Autodesk Fusion 360 part; units mm, degrees
(part 4 of 5)
sketch "Sketch1" plane through (0, 0, 0) normal (0, 0, 1) x (1, 0, 0)
  line L0 (21.55, -50.4796) -> (21.55, -18.7607)
  line L1 (-21.55, -18.7607) -> (-21.55, -50.4796)
  circle A0 centre (15.25, -19.35) radius 2.95 construction
  circle A1 centre (-15.25, -19.35) radius 2.95 construction
  arc A2 (10.3384, 3) -> (6.0958, 1.2426) centre (10.3384, -3) ccw
  line L2 (-27.7114, -5.7461) -> (-23.2215, -12.9316)
  line L3 (29.5877, -66.4969) -> (23.2215, -56.3087)
  arc A3 (21.55, -50.4796) -> (23.2215, -56.3087) centre (32.55, -50.4796) ccw
  line L4 (4.8532, 0) -> (6.0958, 1.2426)
  circle A4 centre (15, -73.65) radius 2.95 construction
  arc A5 (4.5, -61) -> (8.3897, -57.7389) centre (6.3028, -59.2001) ccw
  line L5 (30.5, 15.05) -> (21.55, 15.05)
  arc A6 (8.0447, -57.2462) -> (6.6112, -56.5) centre (6.6112, -58.25) ccw
  line L6 (-4.5, -79.15) -> (4.5, -79.15) construction
  circle A7 centre (30.5, -79.95) radius 2 construction
  circle A8 centre (15.25, -49.85) radius 2.95 construction
  arc A9 (27.3521, -87.3046) -> (36.4601, -74.6136) centre (30.5, -79.95) ccw
  arc A10 (-8.3897, -57.7389) -> (-4.5, -61) centre (-6.3028, -59.2001) ccw
  arc A11 (-30.5, 15.05) -> (-33.9547, -0.1656) centre (-30.5, 7.05) ccw
  arc A12 (-6.0958, 1.2426) -> (-10.3384, 3) centre (-10.3384, -3) ccw
  line L7 (-27.3521, -87.3046) -> (-20.2, -84.2434)
  arc A13 (-31.6483, -69.2394) -> (-29.5877, -66.4969) centre (-46.5487, -55.8985) ccw
  line L8 (-13.5, 3) -> (-10.3384, 3)
  line L9 (-6.0958, 1.2426) -> (-4.8532, 0)
  line L10 (-31.6483, -69.2394) -> (-36.4601, -74.6136)
  arc A14 (15.1961, -0.0598) -> (13.5, 3) centre (13.5, 1) ccw
  arc A15 (19, 46.9161) -> (14.75, 54.55) centre (14.75, 49.55) ccw construction
  arc A16 (-36.4601, -74.6136) -> (-27.3521, -87.3046) centre (-30.5, -79.95) ccw
  circle A17 centre (-15.25, -49.85) radius 2.95 construction
  arc A18 (-6.6112, -56.5) -> (-8.0447, -57.2462) centre (-6.6112, -58.25) ccw
  line L11 (0.3197, 52.9873) -> (5.4482, 50.7517) construction
  arc A19 (2.7973, 58.6708) -> (-2.7973, 58.6708) centre (0, 52.254) ccw construction
  circle A20 centre (-15, -73.65) radius 2.95 construction
  line L12 (-23.2215, -56.3087) -> (-29.5877, -66.4969)
  arc A21 (18.55, 18.05) -> (21.55, 15.05) centre (21.55, 18.05) ccw construction
  arc A22 (-1.3481, 45.8161) -> (1.3481, 45.8161) centre (0, 47.9215) ccw construction
  arc A23 (33.9547, -0.1656) -> (30.5, 15.05) centre (30.5, 7.05) ccw
  line L13 (6.189, -12.7) -> (-6.189, -12.7) construction
  arc A24 (-13.5, 3) -> (-15.1961, -0.0598) centre (-13.5, 1) ccw
  circle A25 centre (15.25, -63.85) radius 1.5
  arc A26 (8.3, -79.15) -> (4.5, -79.15) centre (6.4, -82.51) ccw construction
  circle A27 centre (15.25, 8.95) radius 1.5
  circle A28 centre (-30.5, 7.05) radius 2 construction
  arc A29 (7.55, 40.0871) -> (5.7029, 41.0977) centre (6.35, 40.0871) ccw construction
  arc A30 (9.75, 29.95) -> (11.75, 29.95) centre (10.75, 29.95) ccw construction
  arc A31 (2.35, 33.9294) -> (3.3622, 32.0776) centre (4.55, 33.9294) ccw construction
  line L14 (10.9121, 55.1332) -> (2.7973, 58.6708) construction
  line L15 (-5.4482, 50.7517) -> (-0.3197, 52.9873) construction
  line L16 (9.75, 29.95) -> (9.75, 41.95) construction
  arc A32 (-13.7095, 54.55) -> (-10.9121, 55.1332) centre (-13.7095, 61.55) ccw construction
  line L17 (4.253, 25.5647) -> (8.8217, 22.262) construction
  line L18 (14.75, 54.55) -> (13.7095, 54.55) construction
  line L19 (6.43, 17.6256) -> (2.818, 20.406) construction
  line L20 (-2.7973, 58.6708) -> (-10.9121, 55.1332) construction
  circle A33 centre (-14.75, 49.55) radius 1.5 construction
  line L21 (9.65, 20.6411) -> (9.65, 19.2104) construction
  line L22 (2.35, 33.9294) -> (2.35, 37.7471) construction
  arc A34 (3.3637, 39.5999) -> (2.35, 37.7471) centre (4.55, 37.7471) ccw construction
  line L23 (-8.8217, 22.262) -> (-4.253, 25.5647) construction
  arc A35 (11.75, 41.95) -> (9.75, 41.95) centre (10.75, 41.95) ccw construction
  arc A36 (-13.55, 35.95) -> (-15.55, 35.95) centre (-14.55, 35.95) ccw construction
  line L24 (18.55, 18.05) -> (18.55, 45.3357) construction
  line L25 (-2.35, 24.5922) -> (-2.35, 21.3569) construction
  line L26 (13.55, 23.95) -> (13.55, 35.95) construction
  arc A37 (15.55, 35.95) -> (13.55, 35.95) centre (14.55, 35.95) ccw construction
  circle A38 centre (14.75, 49.55) radius 1.5 construction
  arc A39 (-2.818, 20.406) -> (-2.35, 21.3569) centre (-3.55, 21.3569) ccw construction
  line L27 (7.55, 40.0871) -> (7.55, 33.4162) construction
  arc A40 (5.6227, 48.5531) -> (5.4482, 50.7517) centre (4.9486, 49.6058) ccw construction
  arc A41 (-2.35, 37.7471) -> (-3.3637, 39.5999) centre (-4.55, 37.7471) ccw construction
  arc A42 (-3.3622, 32.0776) -> (-2.35, 33.9294) centre (-4.55, 33.9294) ccw construction
  arc A43 (4.1622, 31.5645) -> (7.55, 33.4162) centre (5.35, 33.4162) ccw construction
  line L28 (-11.75, 29.95) -> (-11.75, 41.95) construction
  line L29 (-2.818, 20.406) -> (-6.43, 17.6256) construction
  line L30 (-9.75, 41.95) -> (-9.75, 29.95) construction
  line L31 (4.1622, 31.5645) -> (3.3622, 32.0776) construction
  arc A44 (-14.75, 54.55) -> (-19, 46.9161) centre (-14.75, 49.55) ccw construction
  line L32 (11.75, 41.95) -> (11.75, 29.95) construction
  line L33 (-13.7095, 54.55) -> (-14.75, 54.55) construction
  line L34 (-15.55, 23.95) -> (-15.55, 35.95) construction
  arc A45 (-15.55, 23.95) -> (-13.55, 23.95) centre (-14.55, 23.95) ccw construction
  line L35 (5.6227, 48.5531) -> (1.3481, 45.8161) construction
  arc A46 (-7.55, 33.4162) -> (-4.1622, 31.5645) centre (-5.35, 33.4162) ccw construction
  line L36 (-9.65, 19.2104) -> (-9.65, 20.6411) construction
  arc A47 (-2.35, 24.5922) -> (-4.253, 25.5647) centre (-3.55, 24.5922) ccw construction
  line L37 (-1.3481, 45.8161) -> (-5.6227, 48.5531) construction
  arc A48 (-5.7029, 41.0977) -> (-7.55, 40.0871) centre (-6.35, 40.0871) ccw construction
  arc A49 (-18.55, 45.3357) -> (-19, 46.9161) centre (-21.55, 45.3357) ccw construction
  line L38 (-3.3622, 32.0776) -> (-4.1622, 31.5645) construction
  arc A50 (4.253, 25.5647) -> (2.35, 24.5922) centre (3.55, 24.5922) ccw construction
  arc A51 (0.3197, 52.9873) -> (-0.3197, 52.9873) centre (0, 52.254) ccw construction
  arc A52 (19, 46.9161) -> (18.55, 45.3357) centre (21.55, 45.3357) ccw construction
  line L39 (2.35, 21.3569) -> (2.35, 24.5922) construction
  arc A53 (10.9121, 55.1332) -> (13.7095, 54.55) centre (13.7095, 61.55) ccw construction
  line L40 (-13.55, 35.95) -> (-13.55, 23.95) construction
  arc A54 (13.55, 23.95) -> (15.55, 23.95) centre (14.55, 23.95) ccw construction
  line L41 (-2.35, 37.7471) -> (-2.35, 33.9294) construction
  line L42 (-7.55, 33.4162) -> (-7.55, 40.0871) construction
  arc A55 (9.65, 20.6411) -> (8.8217, 22.262) centre (7.65, 20.6411) ccw construction
  arc A56 (-5.4482, 50.7517) -> (-5.6227, 48.5531) centre (-4.9486, 49.6058) ccw construction
  arc A57 (2.35, 21.3569) -> (2.818, 20.406) centre (3.55, 21.3569) ccw construction
  arc A58 (-8.8217, 22.262) -> (-9.65, 20.6411) centre (-7.65, 20.6411) ccw construction
  line L43 (-5.7029, 41.0977) -> (-3.3637, 39.5999) construction
  line L44 (3.3637, 39.5999) -> (5.7029, 41.0977) construction
  line L45 (-18.55, 45.3357) -> (-18.55, 18.05) construction
  line L46 (15.55, 35.95) -> (15.55, 23.95) construction
  arc A59 (-9.75, 41.95) -> (-11.75, 41.95) centre (-10.75, 41.95) ccw construction
  arc A60 (-11.75, 29.95) -> (-9.75, 29.95) centre (-10.75, 29.95) ccw construction
  line L47 (4.5, -61) -> (-4.5, -61)
  arc A61 (6.43, 17.6256) -> (9.65, 19.2104) centre (7.65, 19.2104) ccw construction
  arc A62 (-9.65, 19.2104) -> (-6.43, 17.6256) centre (-7.65, 19.2104) ccw construction
  line L48 (36.4601, -74.6136) -> (31.6483, -69.2394)
  arc A63 (-21.55, 15.05) -> (-18.55, 18.05) centre (-21.55, 18.05) ccw construction
  line L49 (-6.6112, -56.5) -> (6.6112, -56.5)
  line L50 (-21.55, 15.05) -> (-30.5, 15.05)
  line L51 (8.0447, -57.2462) -> (8.3897, -57.7389)
  circle A64 centre (-15.25, 8.95) radius 1.5
  line L52 (8.3, -79.15) -> (27.3521, -87.3046) construction
  arc A65 (29.5877, -66.4969) -> (31.6483, -69.2394) centre (46.5487, -55.8985) ccw
  circle A66 centre (-30.5, -79.95) radius 2 construction
  line L53 (-8.3897, -57.7389) -> (-8.0447, -57.2462)
  arc A67 (-27.7114, -5.7461) -> (-33.9547, -0.1656) centre (-40.4322, -13.6949) ccw
  line L54 (10.3384, 3) -> (13.5, 3)
  arc A68 (23.2215, -12.9316) -> (21.55, -18.7607) centre (32.55, -18.7607) ccw
  arc A69 (-23.2215, -56.3087) -> (-21.55, -50.4796) centre (-32.55, -50.4796) ccw
  arc A70 (-4.5, -79.15) -> (-8.3, -79.15) centre (-6.4, -82.51) ccw construction
  arc A71 (33.9547, -0.1656) -> (27.7114, -5.7461) centre (40.4322, -13.6949) ccw
  arc A72 (-21.55, -18.7607) -> (-23.2215, -12.9316) centre (-32.55, -18.7607) ccw
  circle A73 centre (30.5, 7.05) radius 2 construction
  circle A74 centre (-15.25, -63.85) radius 1.5
  line L55 (-4.8532, 0) -> (4.8532, 0)
  line L56 (23.2215, -12.9316) -> (27.7114, -5.7461)
  line L57 (15.1961, -0.0598) -> (9.0119, -10.0491)
  circle A75 centre (-30.5, 7.05) radius 3.375
  circle A76 centre (30.5, 7.05) radius 3.375
  circle A77 centre (-30.5, -79.95) radius 3.375
  circle A78 centre (30.5, -79.95) radius 3.375
  circle A79 centre (-15.25, -19.35) radius 1.5
  circle A80 centre (15.25, -19.35) radius 1.5
  circle A81 centre (15.25, -49.85) radius 1.5
  circle A82 centre (-15.25, -49.85) radius 1.5
  line L58 (-15.25, -19.35) -> (15.25, -49.85) construction
  line L59 (-10, -24.6) -> (10, -24.6) construction
  line L60 (10, -24.6) -> (10, -44.6) construction
  line L61 (10, -44.6) -> (-10, -44.6) construction
  line L62 (-10, -44.6) -> (-10, -24.6) construction
  line L63 (-10, -24.6) -> (10, -44.6) construction
  line L64 (10, -24.6) -> (-10, -44.6) construction
  circle A83 centre (-10, -24.6) radius 1.5
  circle A84 centre (10, -24.6) radius 1.5
  circle A85 centre (10, -44.6) radius 1.5
  circle A86 centre (-10, -44.6) radius 1.5
  circle A87 centre (-15, -73.65) radius 1.5
  circle A88 centre (15, -73.65) radius 1.5
  line L65 (6.189, -11.4) -> (-6.189, -11.4)
  line L66 (0, 44.45) -> (0, -156.9165) construction
  spline S0 degree 5 poles (9.0119, -10.0491) (8.9382, -10.1683) (8.7794, -10.3902) (8.5077, -10.6735) (8.0875, -10.964) (7.4965, -11.2156) (6.9894, -11.3405) (6.5947, -11.3892) (6.3253, -11.4) (6.189, -11.4) knots 0 0 0 0 0 0 0.2 0.4 0.6 0.8 1 1 1 1 1 1
  line L67 (-15.1961, -0.0598) -> (-9.0119, -10.0491)
  spline S1 degree 5 poles (-9.0119, -10.0491) (-8.9382, -10.1683) (-8.7794, -10.3902) (-8.5077, -10.6735) (-8.0875, -10.964) (-7.4965, -11.2156) (-6.9894, -11.3405) (-6.5947, -11.3892) (-6.3253, -11.4) (-6.189, -11.4) knots 0 0 0 0 0 0 0.2 0.4 0.6 0.8 1 1 1 1 1 1
  line L68 (9.2055, -9.7365) -> (8.8184, -10.3617)
  line L69 (6.5567, -11.4) -> (5.8214, -11.4)
  line L70 (-9.2055, -9.7365) -> (-8.8184, -10.3617)
  line L71 (-6.5567, -11.4) -> (-5.8214, -11.4)
  line L72 (-5.45, -16.7) -> (5.45, -16.7)
  line L73 (5.45, -16.7) -> (5.45, -52.5)
  line L74 (5.45, -52.5) -> (-5.45, -52.5)
  line L75 (-5.45, -52.5) -> (-5.45, -16.7)
  line L76 (-5.45, -16.7) -> (5.45, -52.5) construction
  line L77 (5.45, -16.7) -> (-5.45, -52.5) construction
  line L78 (-5.45, -23.1541) -> (-4.312, -16.7)
  line L79 (-5.45, -23.1541) -> (0.7741, -23.1541) construction
  line L80 (-5.45, -46.0459) -> (-4.312, -52.5)
  line L81 (-5.45, -46.0459) -> (1.3736, -46.0459) construction
  line L82 (-4.312, -16.7) -> (-4.312, -52.5) construction
  line L83 (5.45, -46.0459) -> (4.312, -52.5)
  line L84 (5.45, -23.1541) -> (4.312, -16.7)
  line L85 (-20.2, -84.2434) -> (-20.2, -102.0248)
  line L86 (0, 18) -> (5, 18)
  line L87 (21.55, 15.05) -> (9.313, 15.05)
  arc A89 (5, 18) -> (9.313, 15.05) centre (9.313, 19.6778) ccw
  arc A90 (-9.313, 15.05) -> (-5, 18) centre (-9.313, 19.6778) ccw
  line L88 (-21.55, 15.05) -> (-9.313, 15.05)
  line L89 (0, 18) -> (-5, 18)
  line L90 (-15, -73.65) -> (-15, -103.65) construction
  circle A91 centre (-15, -103.65) radius 1.5
  circle A92 centre (-11.5, -118.65) radius 1.5
  circle A93 centre (-11.5, -118.65) radius 4.5
  line L91 (-15.7286, -120.1891) -> (-19.5733, -109.626)
  line L92 (-15.7286, -120.1891) -> (-5.1118, -120.1891) construction
  line L93 (-19.5733, -109.626) -> (-20.2, -102.0248)
  line L94 (0, -116) -> (-7.863, -116)
  line L95 (20.2, -84.2434) -> (20.2, -102.0248)
  circle A94 centre (15, -103.65) radius 1.5
  circle A95 centre (11.5, -118.65) radius 1.5
  line L96 (19.5733, -109.626) -> (20.2, -102.0248)
  line L97 (15.7286, -120.1891) -> (5.1118, -120.1891) construction
  line L98 (15.7286, -120.1891) -> (19.5733, -109.626)
  line L99 (0, -116) -> (7.863, -116)
  circle A96 centre (11.5, -118.65) radius 4.5
  line L100 (0, 44.45) -> (0, -156.9165) construction
  line L101 (27.3521, -87.3046) -> (20.2, -84.2434)
  point P0 (0, 44.45)
  point P1 (0, -34.6)
  point P2 (0, -34.6)
  point P3 (6.4, -82.51)
  point P4 (15, -103.65)
  dimension "d1" = 6.75
  dimension "d2" = 3
  dimension "d3" = 20
  dimension "d4" = 20
  dimension "d5" = 3
  dimension "d6" = 1.3
  dimension "d7" = 10.9
  dimension "d8" = 35.8
  dimension "d9" = 80
  dimension "d10" = 80
  dimension "d12" = 20.2
  dimension "d13" = 5
  dimension "d14" = 18
  dimension "d15" = 30
  dimension "d16" = 15
  dimension "d17" = 11.5
  dimension "d18" = 9
  dimension "d19" = 110
  dimension "d20" = 55
  constraint midpoint L55 origin
  constraint concentric A11 A75
  constraint concentric A23 A76
  constraint concentric A16 A77
  constraint concentric A7 A78
  constraint equal A77 A78
  constraint equal A76 A77
  constraint equal A75 A76
  constraint concentric A1 A79
  constraint concentric A0 A80
  constraint concentric A8 A81
  constraint concentric A17 A82
  constraint equal A81 A82
  constraint equal A80 A81
  constraint equal A79 A80
  constraint coincident A1.centre A79.centre
  constraint coincident A8.centre A81.centre
  constraint horizontal L59
  constraint perpendicular L59 L60
  constraint parallel L59 L61
  constraint parallel L60 L62
  constraint coincident L63 P2
  constraint coincident L64 P2
  constraint midpoint L58 P2
  constraint coincident L59.start L62.end
  constraint coincident L59.end L60.start
  constraint coincident L60.end L61.start
  constraint coincident L61.end L62.start
  constraint equal A85 A86
  constraint equal A84 A85
  constraint equal A83 A84
  constraint concentric A20 A87
  constraint concentric A4 A88
  constraint equal A87 A88
  constraint equal A81 A87
  constraint coincident P0 L66.start
  constraint perpendicular L59 L66
  constraint midpoint L57.end L68
  constraint midpoint L65.start L69
  constraint symmetric A14.start L66 A24.end
  constraint symmetric L57.end L66 L67.end
  constraint symmetric L65.start L66 L65.end
  constraint symmetric L66 L68.start L70.start
  constraint symmetric L66 L68.end L70.end
  constraint symmetric L66 L69.start L71.start
  constraint symmetric L66 L69.end L71.end
  constraint horizontal L72
  constraint perpendicular L72 L73
  constraint parallel L72 L74
  constraint parallel L73 L75
  constraint coincident L76 P2
  constraint coincident L77 P2
  constraint coincident P2 P1
  constraint horizontal L79
  constraint coincident L75 L78.start
  constraint horizontal L81
  constraint coincident L75 L80.start
  constraint coincident L74 L80.end
  constraint vertical L82
  constraint coincident L72 L78.end
  constraint symmetric L66 L78.start L84.start
  constraint symmetric L66 L78.end L84.end
  constraint symmetric L66 L80.start L83.start
  constraint symmetric L66 L80.end L83.end
  constraint parallel L66 L85
  constraint coincident L85 L7.end
  constraint coincident L66 L86.start
  constraint perpendicular L66 L86
  constraint tangent A21 L87
  constraint perpendicular L21 L87
  constraint horizontal L87
  constraint tangent L87 A89
  constraint symmetric L5.end L66 A63.start
  constraint symmetric L66 L86.start L89.start
  constraint symmetric L66 L86.end A90.end
  constraint symmetric L66 L87.end A90.start
  constraint symmetric L66 A89 A90
  constraint coincident A20.centre A87.centre
  constraint vertical L90
  constraint coincident L90.end A91.centre
  constraint equal A87 A91
  constraint equal A91 A92
  constraint concentric A92 A93
  constraint horizontal L92
  constraint coincident A93 L91.start
  constraint tangent A93 L91
  constraint coincident L66 L94.start
  constraint perpendicular L66 L94
  constraint coincident A93 L94.end
  constraint symmetric A70.centre L66 P3
  constraint symmetric P0 L66 L100.start
  constraint symmetric L100.end L66 L66.end
  constraint symmetric L66 L85.end L95.end
  constraint symmetric L66 L7.end L95.start
  constraint symmetric L66 L90.end P4
  constraint symmetric L66 A91 A94
  constraint symmetric L66 A92 A95
  constraint symmetric L66 A93 A96
  constraint symmetric L66 L91.start L97.start
  constraint symmetric L66 L91.end L96.start
  constraint symmetric L66 L92.end L97.end
  constraint symmetric L66 L94.start L99.start
  constraint symmetric L66 L94.end L99.end
  constraint symmetric L7.start L66 A9.start
  measures "d1" diameter of A75
  measures "d2" diameter of A79
  measures "d3" distance of L60.end L61.end
  measures "d4" distance of L59.end L60.end
  measures "d5" diameter of A83
  measures "d7" distance of L73.end L74.end
  measures "d8" distance of L72.end L73.end
  measures "d9" angle of L78 L79
  measures "d10" angle of L80 L81
  measures "d12" distance of L66 L85
  measures "d13" distance of L86.start L86.end
  measures "d14" distance of L55 L86
  measures "d15" distance of A20.centre L90.end
  measures "d16" vertical distance of L90.end A92.centre
  measures "d17" distance of L66 A92.centre
  measures "d18" diameter of A93
  measures "d19" angle of L91 L92
  measures "d20" distance of L47 L94
extrude "Extrude1" add sketch "Sketch1" along normal blind 2 contours L0 L1 L2 L3 A3 L5 A9 A11 L7 A13 L10 A16 L12 A23 L48 L50 A65 A67 A68 A69 A71 A72 L56 L85 L86 L87 A89 A90 L88 L89 A93 L91 L93 L94 L95 L96 L98 L99 A96 L101 | A96 | A93 | L72 L75 L78 | L72 L73 L84 | L74 L75 L80 | L73 L74 L83
fillet "Fillet1" radius 2 2 edges at (-20.2, -84.2434, 1) (20.2, -84.2434, 1)
fillet "Fillet2" radius 4 2 edges at (7.863, -116, 1) (-7.863, -116, 1)
fillet "Fillet3" radius 10 4 edges at (-19.5733, -109.626, 1) (-20.2, -102.0248, 1) (19.5733, -109.626, 1) (20.2, -102.0248, 1)
fillet "Fillet4" radius 1 4 edges at (-4.312, -16.7, 1) (4.312, -16.7, 1) (4.312, -52.5, 1) (-4.312, -52.5, 1)
fillet "Fillet5" radius 10 4 edges at (-5.45, -23.1541, 1) (5.45, -23.1541, 1) (5.45, -46.0459, 1) (-5.45, -46.0459, 1)
sketch "Sketch2" plane through (0, 0, 2) normal (0, 0, 1) x (1, 0, 0)
  arc A0 (20.1662, -102.4349) -> (20.2, -101.6132) centre (10.2, -101.6132) ccw
  line L0 (20.2, -101.6132) -> (20.2, -87.2749)
  arc A1 (22.987, -85.4363) -> (20.2, -87.2749) centre (22.2, -87.2749) ccw
  line L1 (22.987, -85.4363) -> (27.3521, -87.3046)
  arc A2 (27.3521, -87.3046) -> (36.4601, -74.6136) centre (30.5, -79.95) ccw
  line L2 (36.4601, -74.6136) -> (31.6483, -69.2394)
  arc A3 (29.5877, -66.4969) -> (31.6483, -69.2394) centre (46.5487, -55.8985) ccw
  line L3 (29.5877, -66.4969) -> (23.2215, -56.3087)
  arc A4 (21.55, -50.4796) -> (23.2215, -56.3087) centre (32.55, -50.4796) ccw
  line L4 (21.55, -50.4796) -> (21.55, -18.7607)
  arc A5 (23.2215, -12.9316) -> (21.55, -18.7607) centre (32.55, -18.7607) ccw
  line L5 (23.2215, -12.9316) -> (27.7114, -5.7461)
  arc A6 (33.9547, -0.1656) -> (27.7114, -5.7461) centre (40.4322, -13.6949) ccw
  arc A7 (33.9547, -0.1656) -> (30.5, 15.05) centre (30.5, 7.05) ccw
  line L6 (30.5, 15.05) -> (9.313, 15.05)
  arc A8 (5, 18) -> (9.313, 15.05) centre (9.313, 19.6778) ccw
  line L7 (5, 18) -> (-5, 18)
  arc A9 (-9.313, 15.05) -> (-5, 18) centre (-9.313, 19.6778) ccw
  line L8 (-9.313, 15.05) -> (-30.5, 15.05)
  arc A10 (-30.5, 15.05) -> (-33.9547, -0.1656) centre (-30.5, 7.05) ccw
  arc A11 (-27.7114, -5.7461) -> (-33.9547, -0.1656) centre (-40.4322, -13.6949) ccw
  line L9 (-27.7114, -5.7461) -> (-23.2215, -12.9316)
  arc A12 (-21.55, -18.7607) -> (-23.2215, -12.9316) centre (-32.55, -18.7607) ccw
  line L10 (-21.55, -18.7607) -> (-21.55, -50.4796)
  arc A13 (-23.2215, -56.3087) -> (-21.55, -50.4796) centre (-32.55, -50.4796) ccw
  line L11 (-23.2215, -56.3087) -> (-29.5877, -66.4969)
  arc A14 (-31.6483, -69.2394) -> (-29.5877, -66.4969) centre (-46.5487, -55.8985) ccw
  line L12 (-31.6483, -69.2394) -> (-36.4601, -74.6136)
  arc A15 (-36.4601, -74.6136) -> (-27.3521, -87.3046) centre (-30.5, -79.95) ccw
  line L13 (-27.3521, -87.3046) -> (-22.987, -85.4363)
  arc A16 (-20.2, -87.2749) -> (-22.987, -85.4363) centre (-22.2, -87.2749) ccw
  line L14 (-20.2, -87.2749) -> (-20.2, -101.6132)
  arc A17 (-20.2, -101.6132) -> (-20.1662, -102.4349) centre (-10.2, -101.6132) ccw
  line L15 (-20.1662, -102.4349) -> (-19.6835, -108.2886)
  arc A18 (-19.6835, -108.2886) -> (-19.1143, -110.8871) centre (-9.7173, -107.4669) ccw
  line L16 (-19.1143, -110.8871) -> (-15.7286, -120.1891)
  arc A19 (-15.7286, -120.1891) -> (-7.0571, -119.3647) centre (-11.5, -118.65) ccw
  arc A20 (-3.1079, -116) -> (-7.0571, -119.3647) centre (-3.1079, -120) ccw
  line L17 (-3.1079, -116) -> (3.1079, -116)
  arc A21 (7.0571, -119.3647) -> (3.1079, -116) centre (3.1079, -120) ccw
  arc A22 (7.0571, -119.3647) -> (15.7286, -120.1891) centre (11.5, -118.65) ccw
  line L18 (15.7286, -120.1891) -> (19.1143, -110.8871)
  arc A23 (19.1143, -110.8871) -> (19.6835, -108.2886) centre (9.7173, -107.4669) ccw
  line L19 (19.6835, -108.2886) -> (20.1662, -102.4349)
  circle A24 centre (-15.25, -49.85) radius 1.5
  arc A25 (-13.5, 3) -> (-15.1961, -0.0598) centre (-13.5, 1) ccw
  line L20 (-13.5, 3) -> (-10.3384, 3)
  arc A26 (-6.0958, 1.2426) -> (-10.3384, 3) centre (-10.3384, -3) ccw
  line L21 (-6.0958, 1.2426) -> (-4.8532, 0)
  line L22 (-4.8532, 0) -> (4.8532, 0)
  line L23 (4.8532, 0) -> (6.0958, 1.2426)
  arc A27 (10.3384, 3) -> (6.0958, 1.2426) centre (10.3384, -3) ccw
  line L24 (10.3384, 3) -> (13.5, 3)
  arc A28 (15.1961, -0.0598) -> (13.5, 3) centre (13.5, 1) ccw
  line L25 (15.1961, -0.0598) -> (9.0119, -10.0491)
  spline S0 degree 5 poles (9.0119, -10.0491) (8.9382, -10.1683) (8.7794, -10.3902) (8.5077, -10.6735) (8.0875, -10.964) (7.4965, -11.2156) (6.9894, -11.3405) (6.5947, -11.3892) (6.3253, -11.4) (6.189, -11.4) knots 0 0 0 0 0 0 0.2 0.4 0.6 0.8 1 1 1 1 1 1
  line L26 (6.189, -11.4) -> (-6.189, -11.4)
  spline S1 degree 5 poles (-6.189, -11.4) (-6.3253, -11.4) (-6.5947, -11.3892) (-6.9894, -11.3405) (-7.4965, -11.2156) (-8.0875, -10.964) (-8.5077, -10.6735) (-8.7794, -10.3902) (-8.9382, -10.1683) (-9.0119, -10.0491) knots -1 -1 -1 -1 -1 -1 -0.8 -0.6 -0.4 -0.2 0 0 0 0 0 0
  line L27 (-9.0119, -10.0491) -> (-15.1961, -0.0598)
  circle A29 centre (15.25, -49.85) radius 1.5
  circle A30 centre (15.25, -19.35) radius 1.5
  circle A31 centre (-15.25, -19.35) radius 1.5
  circle A32 centre (-15.25, -63.85) radius 1.5
  circle A33 centre (-30.5, 7.05) radius 3.375
  circle A34 centre (15, -73.65) radius 1.5
  circle A35 centre (-15, -73.65) radius 1.5
  circle A36 centre (-10, -44.6) radius 1.5
  circle A37 centre (10, -44.6) radius 1.5
  circle A38 centre (10, -24.6) radius 1.5
  circle A39 centre (-10, -24.6) radius 1.5
  line L28 (5.45, -24.029) -> (5.45, -45.171)
  arc A40 (5.2981, -46.9075) -> (5.45, -45.171) centre (-4.55, -45.171) ccw
  line L29 (5.2981, -46.9075) -> (4.4577, -51.6736)
  arc A41 (3.4729, -52.5) -> (4.4577, -51.6736) centre (3.4729, -51.5) ccw
  line L30 (3.4729, -52.5) -> (-3.4729, -52.5)
  arc A42 (-4.4577, -51.6736) -> (-3.4729, -52.5) centre (-3.4729, -51.5) ccw
  line L31 (-4.4577, -51.6736) -> (-5.2981, -46.9075)
  arc A43 (-5.45, -45.171) -> (-5.2981, -46.9075) centre (4.55, -45.171) ccw
  line L32 (-5.45, -45.171) -> (-5.45, -24.029)
  arc A44 (-5.2981, -22.2925) -> (-5.45, -24.029) centre (4.55, -24.029) ccw
  line L33 (-5.2981, -22.2925) -> (-4.4577, -17.5264)
  arc A45 (-3.4729, -16.7) -> (-4.4577, -17.5264) centre (-3.4729, -17.7) ccw
  line L34 (-3.4729, -16.7) -> (3.4729, -16.7)
  arc A46 (4.4577, -17.5264) -> (3.4729, -16.7) centre (3.4729, -17.7) ccw
  line L35 (4.4577, -17.5264) -> (5.2981, -22.2925)
  arc A47 (5.45, -24.029) -> (5.2981, -22.2925) centre (-4.55, -24.029) ccw
  circle A48 centre (30.5, 7.05) radius 3.375
  circle A49 centre (-30.5, -79.95) radius 3.375
  circle A50 centre (15.25, -63.85) radius 1.5
  circle A51 centre (15.25, 8.95) radius 1.5
  circle A52 centre (-15.25, 8.95) radius 1.5
  arc A53 (4.5, -61) -> (8.3897, -57.7389) centre (6.3028, -59.2001) ccw
  line L36 (4.5, -61) -> (-4.5, -61)
  arc A54 (-8.3897, -57.7389) -> (-4.5, -61) centre (-6.3028, -59.2001) ccw
  line L37 (-8.3897, -57.7389) -> (-8.0447, -57.2462)
  arc A55 (-6.6112, -56.5) -> (-8.0447, -57.2462) centre (-6.6112, -58.25) ccw
  line L38 (-6.6112, -56.5) -> (6.6112, -56.5)
  arc A56 (8.0447, -57.2462) -> (6.6112, -56.5) centre (6.6112, -58.25) ccw
  line L39 (8.0447, -57.2462) -> (8.3897, -57.7389)
  circle A57 centre (30.5, -79.95) radius 3.375
  circle A58 centre (11.5, -118.65) radius 1.5
  circle A59 centre (15, -103.65) radius 1.5
  circle A60 centre (-11.5, -118.65) radius 1.5
  circle A61 centre (-15, -103.65) radius 1.5
  line L40 (0, -116) -> (0, -61) construction
  line L41 (-15, -103.65) -> (-5.1101, -103.65) construction
  circle A62 centre (-10, -103.65) radius 1
  circle A63 centre (-10, -103.65) radius 3
  line L42 (-2.5, -103.3105) -> (-2.5, -113.346)
  line L43 (-2.5, -113.346) -> (-11.1856, -107.81)
  line L44 (-11.1856, -107.81) -> (-11.1856, -106.4058)
  line L45 (-2.5, -103.3105) -> (-4.5464, -101.7117)
  line L46 (-7, -103.65) -> (-7, -103.4617)
  line L47 (-5.25, -101.7117) -> (-4.5464, -101.7117)
  arc A64 (-5.25, -101.7117) -> (-7, -103.4617) centre (-5.25, -103.4617) ccw
  line L48 (-10, -103.65) -> (-10, -83.65) construction
  circle A65 centre (-10, -83.65) radius 1
  circle A66 centre (-10, -83.65) radius 3
  line L49 (-2.5, -84.401) -> (-2.5, -94.9628)
  line L50 (-2.5, -84.401) -> (-5.6804, -81.9162)
  line L51 (-2.5, -84.401) -> (1.142, -84.401) construction
  line L52 (-5.6804, -81.9162) -> (-7.3512, -85.0584)
  line L53 (-9.532, -86.6133) -> (-9.532, -90.422)
  line L54 (-9.532, -90.422) -> (-2.5, -94.9628)
  line L55 (10, -103.65) -> (10, -83.65) construction
  line L56 (2.5, -103.3105) -> (4.5464, -101.7117)
  line L57 (2.5, -103.3105) -> (2.5, -113.346)
  circle A67 centre (10, -103.65) radius 3
  line L58 (2.5, -113.346) -> (11.1856, -107.81)
  circle A68 centre (15, -103.65) radius 1.5
  line L59 (15, -103.65) -> (5.1101, -103.65) construction
  line L60 (11.1856, -107.81) -> (11.1856, -106.4058)
  line L61 (7, -103.65) -> (7, -103.4617)
  circle A69 centre (10, -103.65) radius 1
  line L62 (5.25, -101.7117) -> (4.5464, -101.7117)
  arc A70 (7, -103.4617) -> (5.25, -101.7117) centre (5.25, -103.4617) ccw
  line L63 (9.532, -90.422) -> (2.5, -94.9628)
  line L64 (2.5, -84.401) -> (2.5, -94.9628)
  line L65 (5.6804, -81.9162) -> (7.3512, -85.0584)
  line L66 (2.5, -84.401) -> (-1.142, -84.401) construction
  line L67 (2.5, -84.401) -> (5.6804, -81.9162)
  line L68 (9.532, -86.6133) -> (9.532, -90.422)
  circle A71 centre (10, -83.65) radius 3
  circle A72 centre (10, -83.65) radius 1
  point P0 (10.2, -101.6132)
  point P1 (9.7173, -107.4669)
  dimension "d33" = 2
  dimension "d34" = 5
  dimension "d35" = 6
  dimension "d36" = 2.5
  dimension "d37" = 1.75
  dimension "d38" = 20
  dimension "d39" = 2
  dimension "d40" = 6
  dimension "d41" = 2.5
  dimension "d42" = 128
  dimension "d43" = 142
  dimension "d44" = 80
  constraint midpoint L17 L40.start
  constraint midpoint L36 L40.end
  constraint coincident A61.centre L41.start
  constraint perpendicular L14 L41
  constraint coincident L41 A62.centre
  constraint concentric A62 A63
  constraint parallel L40 L42
  constraint coincident A63 L44.end
  constraint vertical L44
  constraint coincident L41 L46.start
  constraint coincident A63 L46.start
  constraint tangent A63 L46
  constraint perpendicular L46 L47
  constraint tangent L47 A64
  constraint tangent L46 A64
  constraint coincident A62.centre A63.centre
  constraint perpendicular L41 L48
  constraint coincident L48.end A65.centre
  constraint concentric A65 A66
  constraint vertical L49
  constraint horizontal L51
  constraint coincident A66 L52.end
  constraint tangent A66 L52
  constraint coincident A66 L53.start
  constraint parallel L48 L53
  constraint symmetric A17.centre L40 P0
  constraint symmetric A18.centre L40 P1
  constraint symmetric A61 L40 A68
  constraint symmetric L40 A61.centre A59.centre
  constraint symmetric L40 L41.end L59.end
  constraint symmetric L40 A62 A69
  constraint symmetric L40 A63 A67
  constraint symmetric L40 L42.start L56.start
  constraint symmetric L40 L42.end L57.end
  constraint symmetric L40 L43.end L58.end
  constraint symmetric L40 L44.end L60.end
  constraint symmetric L40 L45.end L56.end
  constraint symmetric L40 L46.start L61.start
  constraint symmetric L40 L47.start L62.start
  constraint symmetric L40 L46.end L61.end
  constraint symmetric L40 A64 A70
  constraint symmetric L40 A62.centre L55.start
  constraint symmetric L40 L48.end L55.end
  constraint symmetric L40 A65 A72
  constraint symmetric L40 A66 A71
  constraint symmetric L40 L49.start L64.start
  constraint symmetric L40 L49.end L63.end
  constraint symmetric L40 L50.end L65.start
  constraint symmetric L40 L51.end L66.end
  constraint symmetric L40 L52.end L65.end
  constraint symmetric L40 L53.start L68.start
  constraint symmetric L40 L53.end L63.start
  measures "d33" diameter of A62
  measures "d34" distance of A61.centre A62.centre
  measures "d35" diameter of A63
  measures "d36" distance of L40 L42
  measures "d37" radius of A64
  measures "d38" distance of A62.centre L48.end
  measures "d39" diameter of A65
  measures "d40" diameter of A66
  measures "d41" distance of L40 L49
  measures "d42" angle of L42 L45
  measures "d43" angle of L50 L51
  measures "d44" angle of L50 L52
extrude "Extrude2" cut sketch "Sketch2" against normal blind 2 contours A62 | A63 L42 L43 L44 L45 L46 L47 A64 | A65 | A66 L49 L50 L52 L53 L54 | L56 L57 A67 L58 L60 L61 L62 A70 | A69 | L63 L64 L65 L67 L68 A71 | A72
fillet "Fillet6" radius 2 4 edges at (-5.6804, -81.9162, 1) (-2.5, -84.401, 1) (2.5, -84.401, 1) (5.6804, -81.9162, 1)
fillet "Fillet7" radius 1 4 edges at (-2.5, -94.9628, 1) (2.5, -94.9628, 1) (2.5, -113.346, 1) (-2.5, -113.346, 1)
fillet "Fillet8" radius 1.5 4 edges at (-4.5464, -101.7117, 1) (-2.5, -103.3105, 1) (4.5464, -101.7117, 1) (2.5, -103.3105, 1)
fillet "Fillet9" radius 1.5 4 edges at (-9.532, -90.422, 1) (-9.532, -86.6133, 1) (9.532, -90.422, 1) (9.532, -86.6133, 1)
fillet "Fillet10" radius 1.5 4 edges at (11.1856, -107.81, 1) (11.1856, -106.4058, 1) (-11.1856, -107.81, 1) (-11.1856, -106.4058, 1)
sketch "Sketch3" plane through (0, 0, 2) normal (0, 0, 1) x (1, 0, 0)
  circle A0 centre (10, -103.65) radius 1
  circle A1 centre (-10, -83.65) radius 1
  line L0 (-5.25, -101.7117) -> (-5.0629, -101.7117)
  arc A2 (-4.1394, -102.0297) -> (-5.0629, -101.7117) centre (-5.0629, -103.2117) ccw
  line L1 (-4.1394, -102.0297) -> (-3.0765, -102.8601)
  arc A3 (-2.5, -104.0421) -> (-3.0765, -102.8601) centre (-4, -104.0421) ccw
  line L2 (-2.5, -104.0421) -> (-2.5, -111.5227)
  arc A4 (-4.0375, -112.366) -> (-2.5, -111.5227) centre (-3.5, -111.5227) ccw
  line L3 (-4.0375, -112.366) -> (-9.1581, -109.1022)
  arc A5 (-8.9013, -106.4416) -> (-9.1581, -109.1022) centre (-8.3519, -107.8373) ccw
  arc A6 (-8.9013, -106.4416) -> (-7, -103.65) centre (-10, -103.65) ccw
  line L4 (-7, -103.65) -> (-7, -103.4617)
  arc A7 (-5.25, -101.7117) -> (-7, -103.4617) centre (-5.25, -103.4617) ccw
  line L5 (8.8457, -90.8652) -> (4.0425, -93.9668)
  arc A8 (2.5, -93.1267) -> (4.0425, -93.9668) centre (3.5, -93.1267) ccw
  line L6 (2.5, -93.1267) -> (2.5, -85.3765)
  arc A9 (3.2687, -83.8004) -> (2.5, -85.3765) centre (4.5, -85.3765) ccw
  line L7 (3.2687, -83.8004) -> (3.8022, -83.3836)
  arc A10 (6.7994, -84.0207) -> (3.8022, -83.3836) centre (5.0335, -84.9596) ccw
  line L8 (6.7994, -84.0207) -> (7.3512, -85.0584)
  arc A11 (7.3512, -85.0584) -> (8.688, -86.3479) centre (10, -83.65) ccw
  arc A12 (9.532, -87.6968) -> (8.688, -86.3479) centre (8.032, -87.6968) ccw
  line L9 (9.532, -87.6968) -> (9.532, -89.6051)
  arc A13 (8.8457, -90.8652) -> (9.532, -89.6051) centre (8.032, -89.6051) ccw
  arc A14 (9.1581, -109.1022) -> (8.9013, -106.4416) centre (8.3519, -107.8373) ccw
  line L10 (9.1581, -109.1022) -> (4.0375, -112.366)
  arc A15 (2.5, -111.5227) -> (4.0375, -112.366) centre (3.5, -111.5227) ccw
  line L11 (2.5, -111.5227) -> (2.5, -104.0421)
  arc A16 (3.0765, -102.8601) -> (2.5, -104.0421) centre (4, -104.0421) ccw
  line L12 (3.0765, -102.8601) -> (4.1394, -102.0297)
  arc A17 (5.0629, -101.7117) -> (4.1394, -102.0297) centre (5.0629, -103.2117) ccw
  line L13 (5.0629, -101.7117) -> (5.25, -101.7117)
  arc A18 (7, -103.4617) -> (5.25, -101.7117) centre (5.25, -103.4617) ccw
  line L14 (7, -103.4617) -> (7, -103.65)
  arc A19 (7, -103.65) -> (8.9013, -106.4416) centre (10, -103.65) ccw
  line L15 (-4.0425, -93.9668) -> (-8.8457, -90.8652)
  arc A20 (-9.532, -89.6051) -> (-8.8457, -90.8652) centre (-8.032, -89.6051) ccw
  line L16 (-9.532, -89.6051) -> (-9.532, -87.6968)
  arc A21 (-8.688, -86.3479) -> (-9.532, -87.6968) centre (-8.032, -87.6968) ccw
  arc A22 (-8.688, -86.3479) -> (-7.3512, -85.0584) centre (-10, -83.65) ccw
  line L17 (-7.3512, -85.0584) -> (-6.7994, -84.0207)
  arc A23 (-3.8022, -83.3836) -> (-6.7994, -84.0207) centre (-5.0335, -84.9596) ccw
  line L18 (-3.8022, -83.3836) -> (-3.2687, -83.8004)
  arc A24 (-2.5, -85.3765) -> (-3.2687, -83.8004) centre (-4.5, -85.3765) ccw
  line L19 (-2.5, -85.3765) -> (-2.5, -93.1267)
  arc A25 (-4.0425, -93.9668) -> (-2.5, -93.1267) centre (-3.5, -93.1267) ccw
  circle A26 centre (-10, -103.65) radius 1
  circle A27 centre (10, -83.65) radius 1
  arc A28 (20.1662, -102.4349) -> (20.2, -101.6132) centre (10.2, -101.6132) ccw
  line L20 (20.2, -101.6132) -> (20.2, -87.2749)
  arc A29 (22.987, -85.4363) -> (20.2, -87.2749) centre (22.2, -87.2749) ccw
  line L21 (22.987, -85.4363) -> (27.3521, -87.3046)
  arc A30 (27.3521, -87.3046) -> (36.4601, -74.6136) centre (30.5, -79.95) ccw
  line L22 (36.4601, -74.6136) -> (31.6483, -69.2394)
  arc A31 (29.5877, -66.4969) -> (31.6483, -69.2394) centre (46.5487, -55.8985) ccw
  line L23 (29.5877, -66.4969) -> (23.2215, -56.3087)
  arc A32 (21.55, -50.4796) -> (23.2215, -56.3087) centre (32.55, -50.4796) ccw
  line L24 (21.55, -50.4796) -> (21.55, -18.7607)
  arc A33 (23.2215, -12.9316) -> (21.55, -18.7607) centre (32.55, -18.7607) ccw
  line L25 (23.2215, -12.9316) -> (27.7114, -5.7461)
  arc A34 (33.9547, -0.1656) -> (27.7114, -5.7461) centre (40.4322, -13.6949) ccw
  arc A35 (33.9547, -0.1656) -> (30.5, 15.05) centre (30.5, 7.05) ccw
  line L26 (30.5, 15.05) -> (9.313, 15.05)
  arc A36 (5, 18) -> (9.313, 15.05) centre (9.313, 19.6778) ccw
  line L27 (5, 18) -> (-5, 18)
  arc A37 (-9.313, 15.05) -> (-5, 18) centre (-9.313, 19.6778) ccw
  line L28 (-9.313, 15.05) -> (-30.5, 15.05)
  arc A38 (-30.5, 15.05) -> (-33.9547, -0.1656) centre (-30.5, 7.05) ccw
  arc A39 (-27.7114, -5.7461) -> (-33.9547, -0.1656) centre (-40.4322, -13.6949) ccw
  line L29 (-27.7114, -5.7461) -> (-23.2215, -12.9316)
  arc A40 (-21.55, -18.7607) -> (-23.2215, -12.9316) centre (-32.55, -18.7607) ccw
  line L30 (-21.55, -18.7607) -> (-21.55, -50.4796)
  arc A41 (-23.2215, -56.3087) -> (-21.55, -50.4796) centre (-32.55, -50.4796) ccw
  line L31 (-23.2215, -56.3087) -> (-29.5877, -66.4969)
  arc A42 (-31.6483, -69.2394) -> (-29.5877, -66.4969) centre (-46.5487, -55.8985) ccw
  line L32 (-31.6483, -69.2394) -> (-36.4601, -74.6136)
  arc A43 (-36.4601, -74.6136) -> (-27.3521, -87.3046) centre (-30.5, -79.95) ccw
  line L33 (-27.3521, -87.3046) -> (-22.987, -85.4363)
  arc A44 (-20.2, -87.2749) -> (-22.987, -85.4363) centre (-22.2, -87.2749) ccw
  line L34 (-20.2, -87.2749) -> (-20.2, -101.6132)
  arc A45 (-20.2, -101.6132) -> (-20.1662, -102.4349) centre (-10.2, -101.6132) ccw
  line L35 (-20.1662, -102.4349) -> (-19.6835, -108.2886)
  arc A46 (-19.6835, -108.2886) -> (-19.1143, -110.8871) centre (-9.7173, -107.4669) ccw
  line L36 (-19.1143, -110.8871) -> (-15.7286, -120.1891)
  arc A47 (-15.7286, -120.1891) -> (-7.0571, -119.3647) centre (-11.5, -118.65) ccw
  arc A48 (-3.1079, -116) -> (-7.0571, -119.3647) centre (-3.1079, -120) ccw
  line L37 (-3.1079, -116) -> (3.1079, -116)
  arc A49 (7.0571, -119.3647) -> (3.1079, -116) centre (3.1079, -120) ccw
  arc A50 (7.0571, -119.3647) -> (15.7286, -120.1891) centre (11.5, -118.65) ccw
  line L38 (15.7286, -120.1891) -> (19.1143, -110.8871)
  arc A51 (19.1143, -110.8871) -> (19.6835, -108.2886) centre (9.7173, -107.4669) ccw
  line L39 (19.6835, -108.2886) -> (20.1662, -102.4349)
  circle A52 centre (-15.25, -49.85) radius 1.5
  arc A53 (-13.5, 3) -> (-15.1961, -0.0598) centre (-13.5, 1) ccw
  line L40 (-13.5, 3) -> (-10.3384, 3)
  arc A54 (-6.0958, 1.2426) -> (-10.3384, 3) centre (-10.3384, -3) ccw
  line L41 (-6.0958, 1.2426) -> (-4.8532, 0)
  line L42 (-4.8532, 0) -> (4.8532, 0)
  line L43 (4.8532, 0) -> (6.0958, 1.2426)
  arc A55 (10.3384, 3) -> (6.0958, 1.2426) centre (10.3384, -3) ccw
  line L44 (10.3384, 3) -> (13.5, 3)
  arc A56 (15.1961, -0.0598) -> (13.5, 3) centre (13.5, 1) ccw
  line L45 (15.1961, -0.0598) -> (9.0119, -10.0491)
  spline S0 degree 5 poles (9.0119, -10.0491) (8.9382, -10.1683) (8.7794, -10.3902) (8.5077, -10.6735) (8.0875, -10.964) (7.4965, -11.2156) (6.9894, -11.3405) (6.5947, -11.3892) (6.3253, -11.4) (6.189, -11.4) knots 0 0 0 0 0 0 0.2 0.4 0.6 0.8 1 1 1 1 1 1
  line L46 (6.189, -11.4) -> (-6.189, -11.4)
  spline S1 degree 5 poles (-6.189, -11.4) (-6.3253, -11.4) (-6.5947, -11.3892) (-6.9894, -11.3405) (-7.4965, -11.2156) (-8.0875, -10.964) (-8.5077, -10.6735) (-8.7794, -10.3902) (-8.9382, -10.1683) (-9.0119, -10.0491) knots -1 -1 -1 -1 -1 -1 -0.8 -0.6 -0.4 -0.2 0 0 0 0 0 0
  line L47 (-9.0119, -10.0491) -> (-15.1961, -0.0598)
  circle A57 centre (15.25, -49.85) radius 1.5
  circle A58 centre (15.25, -19.35) radius 1.5
  circle A59 centre (-15.25, -19.35) radius 1.5
  circle A60 centre (-15.25, -63.85) radius 1.5
  circle A61 centre (-30.5, 7.05) radius 3.375
  circle A62 centre (15, -73.65) radius 1.5
  circle A63 centre (-15, -73.65) radius 1.5
  circle A64 centre (-10, -44.6) radius 1.5
  circle A65 centre (10, -44.6) radius 1.5
  circle A66 centre (10, -24.6) radius 1.5
  circle A67 centre (-10, -24.6) radius 1.5
  line L48 (5.45, -24.029) -> (5.45, -45.171)
  arc A68 (5.2981, -46.9075) -> (5.45, -45.171) centre (-4.55, -45.171) ccw
  line L49 (5.2981, -46.9075) -> (4.4577, -51.6736)
  arc A69 (3.4729, -52.5) -> (4.4577, -51.6736) centre (3.4729, -51.5) ccw
  line L50 (3.4729, -52.5) -> (-3.4729, -52.5)
  arc A70 (-4.4577, -51.6736) -> (-3.4729, -52.5) centre (-3.4729, -51.5) ccw
  line L51 (-4.4577, -51.6736) -> (-5.2981, -46.9075)
  arc A71 (-5.45, -45.171) -> (-5.2981, -46.9075) centre (4.55, -45.171) ccw
  line L52 (-5.45, -45.171) -> (-5.45, -24.029)
  arc A72 (-5.2981, -22.2925) -> (-5.45, -24.029) centre (4.55, -24.029) ccw
  line L53 (-5.2981, -22.2925) -> (-4.4577, -17.5264)
  arc A73 (-3.4729, -16.7) -> (-4.4577, -17.5264) centre (-3.4729, -17.7) ccw
  line L54 (-3.4729, -16.7) -> (3.4729, -16.7)
  arc A74 (4.4577, -17.5264) -> (3.4729, -16.7) centre (3.4729, -17.7) ccw
  line L55 (4.4577, -17.5264) -> (5.2981, -22.2925)
  arc A75 (5.45, -24.029) -> (5.2981, -22.2925) centre (-4.55, -24.029) ccw
  circle A76 centre (30.5, 7.05) radius 3.375
  circle A77 centre (-30.5, -79.95) radius 3.375
  circle A78 centre (15.25, -63.85) radius 1.5
  circle A79 centre (15.25, 8.95) radius 1.5
  circle A80 centre (-15.25, 8.95) radius 1.5
  arc A81 (4.5, -61) -> (8.3897, -57.7389) centre (6.3028, -59.2001) ccw
  line L56 (4.5, -61) -> (-4.5, -61)
  arc A82 (-8.3897, -57.7389) -> (-4.5, -61) centre (-6.3028, -59.2001) ccw
  line L57 (-8.3897, -57.7389) -> (-8.0447, -57.2462)
  arc A83 (-6.6112, -56.5) -> (-8.0447, -57.2462) centre (-6.6112, -58.25) ccw
  line L58 (-6.6112, -56.5) -> (6.6112, -56.5)
  arc A84 (8.0447, -57.2462) -> (6.6112, -56.5) centre (6.6112, -58.25) ccw
  line L59 (8.0447, -57.2462) -> (8.3897, -57.7389)
  circle A85 centre (30.5, -79.95) radius 3.375
  circle A86 centre (11.5, -118.65) radius 1.5
  circle A87 centre (15, -103.65) radius 1.5
  circle A88 centre (-11.5, -118.65) radius 1.5
  circle A89 centre (-15, -103.65) radius 1.5
equation "d6 = 12.7 mm - 11.4 mm"
equation "d12 = ( 40.4 / 2 ) * 1 mm"
equation "d17 = ( 23 / 2 ) * 1 mm"
equation "d34 = 2.5 mm + 1 mm + 1.5 mm"

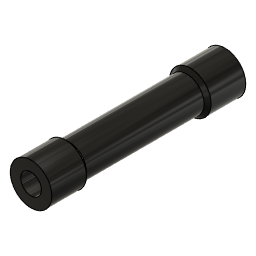
design "m3_standoff_28mm"
Autodesk Fusion 360 part; units mm, degrees
sketch "Sketch1" plane through (0, 0, 0) normal (0, 1, 0) x (1, 0, 0)
  line L0 (0, 0) -> (0, 28) construction
  line L1 (0, 28) -> (1.5, 28)
  line L2 (1.5, 28) -> (1.5, 0)
  line L3 (1.5, 0) -> (0, 0)
  line L4 (0, 0) -> (0, 28)
  line L5 (0, 28) -> (3, 28)
  line L6 (3, 28) -> (3, 23)
  line L7 (3, 23) -> (0, 23)
  line L8 (0, 23) -> (0, 28)
  line L9 (0, 0) -> (3, 0)
  line L10 (3, 0) -> (3, 5)
  line L11 (3, 5) -> (0, 5)
  line L12 (0, 5) -> (0, 0)
  line L13 (0, 23) -> (2.5, 23)
  line L14 (2.5, 23) -> (2.5, 5)
  line L15 (2.5, 5) -> (0, 5)
  line L16 (0, 5) -> (0, 23)
  dimension "d1" = 28
  dimension "d2" = 1.5
  dimension "d3" = 28
  dimension "d4" = 3
  dimension "d5" = 5
  dimension "d6" = 3
  dimension "d7" = 5
  dimension "d8" = 2.5
  constraint coincident L0.start L3.end
  constraint vertical L0
  constraint horizontal L1
  constraint vertical L2
  constraint horizontal L3
  constraint vertical L4
  constraint horizontal L5
  constraint vertical L6
  constraint horizontal L7
  constraint vertical L8
  constraint horizontal L9
  constraint vertical L10
  constraint horizontal L11
  constraint vertical L12
  constraint horizontal L13
  constraint vertical L14
  constraint horizontal L15
  constraint vertical L16
  measures "d1" distance of L0.start L0.end
  measures "d2" distance of L0.end L1.end
  measures "d3" distance of L0.end L0.start
  measures "d4" distance of L0.end L5.end
  measures "d5" distance of L0.end L7.end
  measures "d6" distance of L0.start L9.end
  measures "d7" distance of L0.start L11.end
  measures "d8" distance of L7.end L13.end
revolve "Revolve1" add sketch "Sketch1" angle 360 about axis through (0, 0, -5) along (0, 0, -1) contours L2 L5 L6 L7 L13 | L2 L7 L11 L13 L14 L15 | L2 L9 L10 L11 L15
chamfer "Chamfer1" distance 0.5 angle 45 2 edges at (-2.3308, -0.904, -23) (-2.3308, -0.904, -5)

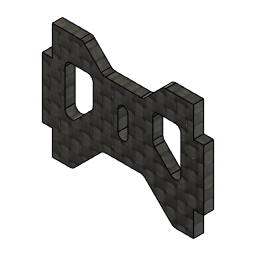
design "cam_mount_2mm"
Autodesk Fusion 360 part; units mm, degrees
sketch "Sketch1" plane through (0, 0, 0) normal (0, 0, 1) x (1, 0, 0)
  line L0 (-16, 11.5) -> (16, 11.5)
  line L1 (16, 11.5) -> (16, -11.5)
  line L2 (16, -11.5) -> (-16, -11.5)
  line L3 (-16, -11.5) -> (-16, 11.5)
  line L4 (-16, 11.5) -> (16, -11.5) construction
  line L5 (16, 11.5) -> (-16, -11.5) construction
  dimension "d1" = 32
  dimension "d2" = 23
  constraint horizontal L0
  constraint perpendicular L0 L1
  constraint parallel L0 L2
  constraint parallel L1 L3
  constraint coincident L4 origin
  constraint coincident L5 origin
  measures "d1" distance of L1.end L2.end
  measures "d2" distance of L0.end L1.end
sketch "Sketch2" plane through (0, 0, 0) normal (0, 0, 1) x (1, 0, 0)
  line L0 (-14, 11.5) -> (14, 11.5)
  line L1 (14, 11.5) -> (14, -11.5)
  line L2 (14, -11.5) -> (-14, -11.5)
  line L3 (-14, -11.5) -> (-14, 11.5)
  line L4 (-14, 11.5) -> (14, -11.5) construction
  line L5 (14, 11.5) -> (-14, -11.5) construction
  line L6 (-16, 5.5) -> (-14, 5.5)
  line L7 (-14, 5.5) -> (-14, -6.5)
  line L8 (-14, -6.5) -> (-16, -6.5)
  line L9 (-16, -6.5) -> (-16, 5.5)
  line L10 (-16, -11.5) -> (-16, 11.5)
  line L11 (-4, 7.5) -> (4, 7.5)
  line L12 (-16, 11.5) -> (16, 11.5)
  line L13 (-4, 7.5) -> (-8, 11.5)
  line L14 (-4, 7.5) -> (0.1526, 7.5) construction
  line L15 (4, 7.5) -> (8, 11.5)
  line L16 (4, 7.5) -> (8.8443, 7.5) construction
  line L17 (0, 0) -> (0, 17.5574) construction
  line L18 (-4, -5.5) -> (4, -5.5)
  line L19 (-4, -5.5) -> (-10, -11.5)
  line L20 (-4, -5.5) -> (4.4853, -5.5) construction
  line L21 (4, -5.5) -> (10, -11.5)
  line L22 (14, 5.5) -> (16, 5.5)
  line L23 (16, 5.5) -> (16, -6.5)
  line L24 (16, -6.5) -> (14, -6.5)
  line L25 (14, -6.5) -> (14, 5.5)
  line L26 (16, 11.5) -> (16, -11.5)
  line L27 (-1, 3.3) -> (-1, -0.7)
  arc A0 (-1, -0.7) -> (1, -0.7) centre (0, -0.7) ccw
  line L28 (1, -0.7) -> (1, 3.3)
  arc A1 (1, 3.3) -> (-1, 3.3) centre (0, 3.3) ccw
  line L29 (0, 4.3) -> (0, -1.7) construction
  line L30 (11.5, 6.5) -> (5.9, 6.5)
  line L31 (5.9, 6.5) -> (5.9, -2.8)
  line L32 (5.9, -2.8) -> (11.5, -2.8)
  line L33 (11.5, -2.8) -> (11.5, 6.5)
  line L34 (5.9, 0.7355) -> (9.4355, -2.8)
  line L35 (5.9, 0.7355) -> (4.4836, 0.7355) construction
  line L36 (11.5, -2.8) -> (11.5, -4.8645)
  line L37 (11.5, -4.8645) -> (9.4355, -2.8)
  point P0 (0, 7.5)
  dimension "d3" = 28
  dimension "d4" = 23
  dimension "d5" = 12
  dimension "d6" = 4
  dimension "d7" = 135
  dimension "d8" = 45
  dimension "d9" = 8
  dimension "d10" = 13
  dimension "d11" = 135
  dimension "d12" = 90
  dimension "d13" = 6
  dimension "d14" = 12
  dimension "d15" = 6
  dimension "d16" = 2
  dimension "d17" = 6
  dimension "d18" = 3.8
  dimension "d19" = 5.6
  dimension "d20" = 9.3
  dimension "d21" = 2.5
  dimension "d22" = 1
  dimension "d23" = 45
  dimension "d24" = 5
  constraint horizontal L0
  constraint perpendicular L0 L1
  constraint parallel L0 L2
  constraint parallel L1 L3
  constraint coincident L4 L17.start
  constraint coincident L5 L17.start
  constraint coincident L17.start origin
  constraint horizontal L6
  constraint vertical L7
  constraint horizontal L8
  constraint vertical L9
  constraint coincident L3 L7.end
  constraint coincident L6.start L10
  constraint horizontal L11
  constraint horizontal L14
  constraint coincident L0 L13.end
  constraint horizontal L16
  constraint coincident L0 L15.end
  constraint vertical L17
  constraint midpoint L11 P0
  constraint coincident L17 P0
  constraint horizontal L20
  constraint coincident L2 L19.end
  constraint coincident L2 L21.end
  constraint horizontal L22
  constraint vertical L23
  constraint horizontal L24
  constraint vertical L25
  constraint coincident L1 L22.start
  constraint coincident L22.end L26
  constraint tangent L27 A0
  constraint tangent A0 L28
  constraint parallel L27 L28
  constraint tangent L28 A1
  constraint tangent L27 A1
  constraint midpoint A1 L29.start
  constraint midpoint A0 L29.end
  constraint parallel L17 L29
  constraint coincident L17 L29.start
  constraint horizontal L30
  constraint vertical L31
  constraint horizontal L32
  constraint vertical L33
  constraint horizontal L35
  constraint coincident L31 L34.start
  constraint coincident L32 L34.end
  constraint perpendicular L32 L36
  constraint parallel L34 L37
  measures "d3" distance of L1.end L2.end
  measures "d4" distance of L0.end L1.end
  measures "d5" distance of L6 L8
  measures "d6" distance of L11 L12
  measures "d7" angle of L13 L14
  measures "d8" angle of L15 L16
  measures "d9" distance of L11.start L11.end
  measures "d11" angle of L19 L20
  measures "d12" angle of L19 L21
  measures "d13" distance of L6 L12
  measures "d14" distance of L22.start L24.end
  measures "d15" distance of L12 L22
  measures "d16" diameter of A0
  measures "d17" distance of L29.start L29.end
  measures "d18" distance of L20 L29.end
  measures "d19" distance of L30.start L30.end
  measures "d20" distance of L30.start L32.end
  measures "d21" distance of L25 L33
  measures "d22" distance of L11 L30
  measures "d23" angle of L34 L35
  measures "d24" distance of L34.start L34.end
extrude "Extrude1" add sketch "Sketch2" along normal blind 2 contours L0 L1 L2 L3 L7 L11 L12 L13 L15 L18 L19 L21 L25 | L3 L6 L7 L8 L9 L10 | L1 L22 L23 L24 L25 L26 | L30 L31 L32 L33 L34 | L32 L36 L37 | L31 L32 L34
extrude "Extrude2" cut sketch "Sketch2" along normal blind 5 contours L30 L31 L32 L33 L34 | L32 L36 L37
fillet "Fillet1" radius 1.2 4 edges at (11.5, -4.8645, 1) (5.9, 0.7355, 1) (5.9, 6.5, 1) (11.5, 6.5, 1)
mirror "Mirror1" about plane through (0, 0, 0) normal (1, 0, 0) of "Extrude2", "Fillet1"
fillet "Fillet2" radius 1.2 8 edges at (-4, -5.5, 1) (-10, -11.5, 1) (4, -5.5, 1) (10, -11.5, 1) (-8, 11.5, 1) (-4, 7.5, 1) (4, 7.5, 1) (8, 11.5, 1)

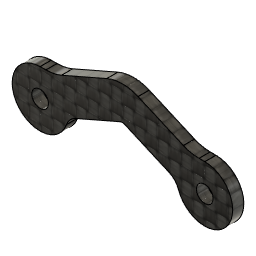
design "nose_protect"
Autodesk Fusion 360 part; units mm, degrees